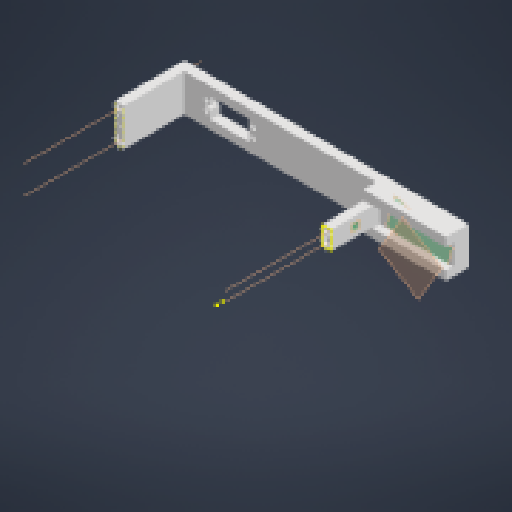
# Autodesk Inventor part: Main Rail
Saved by Autodesk Inventor 2025.2 (Build 292293000, 293)
## iProperties
Created: 2024-11-17
Part Number: Main Rail
Material: Generic
Document SubType Name: Modeling
Designer: JL
Density: 1 g/cm^3
Appearance: Default
Author: JL
Autodesk Inventor part; units mm, degrees
ref_plane "Work Plane1" through (160.0305, 116.6136, -77.6157) normal (0, 0, -1) x (-0.9606716, 0.277687, 0)
ref_plane "Work Plane3" through (116.7456, 115.7996, -51.6157) normal (-1, 0, 0) x (0, 0, 1)
ref_plane "Work Plane2" through (114.2456, 115.7996, -51.6157) normal (-1, 0, 0) x (0, 0, 1)
sketch "Sketch3" plane through (116.7456, 115.7996, -51.6157) normal (-1, 0, 0) x (0, 0, 1)
  circle A0 centre (0, 0) radius 4 construction
  line L0 (-26, 10) -> (0, 10)
  line L1 (0, 10) -> (0, -10)
  line L2 (0, -10) -> (-26, -10)
  line L3 (-26, -10) -> (-26, 10) projected
  point P0 (51.6157, -115.7996)
  constraints: 6 end point, 2 perpendicular, 1 horizontal, 1 midpoint
extrude "Extrusion3" add sketch "Sketch3" along normal blind 10
ref_plane "Work Plane4" through (185.8339, 132.1316, -51.6157) normal (0, 0, 1) x (-0.8564988, 0.516149, 0)
mirror "Mirror1" about plane through (185.8339, 132.1316, -51.6157) normal (0, 0, 1) of "Extrusion3"
sketch "Sketch4" plane through (116.7456, 115.7996, -51.6157) normal (1, 0, 0) x (0, 0, -1)
  circle A0 centre (0, 0) radius 4 projected
  point P0 (-51.6157, -115.7996)
extrude "Extrusion4" cut sketch "Sketch4" against normal up to surface (2.5 mm away)
ref_plane "Work Plane6" through (-26.356, 110.799, -94.8157) normal (0, 0, -1) x (0.8545404, 0.519385, 0)
sketch "Sketch7" plane through (116.7456, 105.7996, -25.6157) normal (0, 0, 1) x (1, 0, 0)
  line L0 (0, 20) -> (0, 0) projected
  line L1 (0, 20) -> (-10, 20) projected
  line L2 (-10, 20) -> (-10, 0) projected
  line L3 (0, 0) -> (-10, 0) projected
  line L4 (0, 10) -> (-10, 10) construction
  line L5 (-5, 10) -> (-5, 0) construction
  point P0 (-116.7456, -105.7996)
  point P1 (-5, 5)
  point P2 (-5, 15)
  constraints: 5 midpoint, 4 end point, 1 symmetric about line
sketch "Sketch11" plane through (-26.356, 110.799, -94.8157) normal (0, 0, -1) x (0.8545404, 0.519385, 0)
  line L0 (4.1262, -15.4557) -> (-6.6251, 2.2333) construction
  line L1 (-6.6251, 2.2333) -> (-41.9176, -19.2173) construction
  line L2 (-41.9176, -19.2173) -> (-31.1663, -36.9063) construction
  line L3 (-31.1663, -36.9063) -> (4.1262, -15.4557) construction
  line L4 (147.168, 71.8939) -> (180.9407, 92.4208) construction
  line L5 (170.553, 109.5116) -> (136.7803, 88.9847) construction
  line L6 (17.8654, -18.8072) -> (-3.2735, 15.9725) construction
  line L7 (-3.2735, 15.9725) -> (-55.6569, -15.8658)
  line L8 (-55.6569, -15.8658) -> (-34.5179, -50.6455) construction
  line L9 (-34.5179, -50.6455) -> (17.8654, -18.8072)
  line L10 (180.9407, 92.4208) -> (198.0315, 102.8085) construction
  line L11 (198.0315, 102.8085) -> (187.4621, 120.1984)
  line L12 (187.6438, 119.8993) -> (170.553, 109.5116) construction
  line L13 (17.8654, -18.8072) -> (203.4072, 93.964)
  line L14 (203.4072, 93.964) -> (198.0315, 102.8085)
  line L15 (187.4621, 120.1984) -> (182.2682, 128.7438)
  line L16 (182.2682, 128.7438) -> (-3.2735, 15.9725)
  circle A0 centre (-27.3984, -22.5044) radius 24.5216 construction
  line L17 (-48.3531, -35.2405) -> (-69.7166, -48.2251) construction
  line L18 (-34.5179, -50.6455) -> (-59.1471, -65.615)
  line L19 (-59.1471, -65.615) -> (-80.2861, -30.8352)
  line L20 (-80.2861, -30.8352) -> (-55.6569, -15.8658)
  line L21 (-42.6046, -19.0497) -> (-6.4575, 2.9203)
  line L22 (-6.4575, 2.9203) -> (4.8131, -15.6233)
  line L23 (4.8131, -15.6233) -> (-31.3339, -37.5933)
  line L24 (-31.3339, -37.5933) -> (-42.6046, -19.0497)
  point P0 (-35.0251, 108.3711)
  dimension "d31" = 10
  dimension "d32" = 20
  dimension "d33" = 25
  dimension "d34" = 0.5
  constraints: 38 end point, 5 perpendicular, 3 collinear, 3 point on line, 1 midpoint, 1 parallel, 9 other
  measures "d31" distance between parallel lines of L3 L9
  measures "d32" distance of L4.end L10.end
  measures "d33" distance of L17.end L17.start
  measures "d34" distance between parallel lines of L1 L21
ref_plane "Work Plane7" through (-30.7879, 116.4111, -84.2157) normal (0, 0, 1) x (0.7646407, 0.6444568, 0)
extrude "Extrusion8" add sketch "Sketch11" against normal up to surface (10.6 mm away)
sketch "Sketch12" plane through (-110.979, 136.1496, -84.2157) normal (0, 0, 1) x (1, 0, 0)
  line L0 (217.7246, -10.35) -> (217.7246, -30.35) projected
  line L1 (307.2462, 0) -> (307.2462, -40.7) projected
  line L2 (0, 0) -> (307.2462, 0) projected
  line L3 (0, -40.7) -> (0, 0) projected
  line L4 (307.2462, -40.7) -> (0, -40.7) projected
  line L5 (217.7246, -10.35) -> (217.7246, 0)
  line L6 (0, 0) -> (307.2462, 0) projected
  line L7 (217.7246, -30.35) -> (217.7246, -40.7)
  point P0 (110.979, -136.1496)
  point P1 (217.7246, 0)
  constraints: 4 end point, 3 point on line, 1 perpendicular
extrude "Extrusion9" add sketch "Sketch12" along normal up to surface (6.6 mm away) contours L5 L2 L1 L4 L7 L0
sketch "Sketch13" plane through (116.7456, 105.7996, -77.6157) normal (0, 0, 1) x (1, 0, 0)
  line L0 (0, 0) -> (-10, 0) projected
  line L1 (-10, 0) -> (-10, -10.35) projected
  line L2 (-10, -10.35) -> (79.5216, -10.35) projected
  line L3 (79.5216, -10.35) -> (79.5216, 30.35) projected
  line L4 (79.5216, 30.35) -> (-10, 30.35) projected
  line L5 (-10, 30.35) -> (-10, 20) projected
  line L6 (0, 20) -> (-10, 20) projected
  line L7 (0, 20) -> (0, 0) projected
  line L8 (0, 20) -> (79.5216, 20)
  line L9 (0, 0) -> (79.5216, 0)
  point P0 (-116.7456, -105.7996)
  constraints: 4 end point, 2 perpendicular, 2 point on line
extrude "Extrusion10" add sketch "Sketch13" along normal blind 7.5 contours L9 L3 L2 L1 L0 | L6 L5 L4 L3 L8
sketch "Sketch14" plane through (-110.979, 136.1496, -84.2157) normal (0, 0, 1) x (1, 0, 0)
  line L0 (0, 0) -> (307.2462, 0) projected
  line L1 (307.2462, -40.7) -> (0, -40.7) projected
  line L2 (0, 0) -> (10, 0)
  line L3 (10, 0) -> (10, -40.7)
  line L4 (10, -40.7) -> (0, -40.7)
  line L5 (0, -40.7) -> (0, 0)
  point P0 (110.979, -136.1496)
  point P1 (10, 0)
  dimension "d41" = 10
  constraints: 8 end point, 2 parallel, 1 horizontal, 1 perpendicular, 1 point on line
  measures "d41" distance between parallel lines of L5 L3
extrude "Extrusion11" add sketch "Sketch14" along normal up to surface (32.6 mm away)
mirror "Mirror2" about plane through (185.8339, 132.1316, -51.6157) normal (0, 0, 1) of "Extrusion11"
sketch "Sketch15" plane through (-110.979, 95.4496, -19.0157) normal (0, 0, 1) x (1, 0, 0)
  line L0 (0, 0) -> (10, 0) construction
  line L1 (5, 0) -> (5, 10) construction
  line L2 (10, 0) -> (10, 40.7) construction
  line L3 (10, 20.35) -> (0, 20.35) construction
  line L4 (0, 40.7) -> (0, 0) construction
  point P0 (110.979, -95.4496)
  point P1 (5, 5)
  point P2 (5, 35.7)
  constraints: 4 end point, 4 midpoint, 1 perpendicular, 1 symmetric about line, 1 vertical
sketch "Sketch17" plane through (116.7456, 105.7996, -25.6157) normal (0, 0, 1) x (1, 0, 0)
  circle A0 centre (-5.0015, 4.9996) radius 2.77 projected
  circle A1 centre (-5.0015, 14.9996) radius 2.77 projected
  point P0 (-116.7456, -105.7996)
ref_plane "Work Plane10" through (108.2326, 107.2877, -33.7157) normal (0, 0, -1) x (0.3976268, 0.9175472, 0)
extrude "Extrusion13" cut sketch "Sketch17" against normal up to surface (8.1 mm away)
sketch "Sketch18" plane through (111.7441, 110.7992, -33.7157) normal (0, 0, 1) x (1, 0, 0)
  circle A0 centre (0, 0) radius 2.77 projected
  circle A1 centre (0, 10) radius 2.77 projected
  point P0 (-111.7441, -110.7992)
  constraints: 2 coincident
hole "Hole2" at (111.7441, 110.7992, -33.7157) at (111.7441, 120.7992, -33.7157) direction (0, 0, -1) diameter 4.3 end through all clearance for "Flat Head Machine Screw" size "M4" standard "Ansi Metric M Profile"
sketch "Sketch19" plane through (-110.979, 95.4496, -19.0157) normal (0, 0, 1) x (1, 0, 0)
  circle A0 centre (4.9984, 35.7) radius 2.77 projected
  circle A1 centre (4.9985, 4.9996) radius 2.77 projected
  point P0 (110.979, -95.4496)
ref_plane "Work Plane11" through (-109.4921, 96.9377, -27.1157) normal (0, 0, -1) x (0.3976268, 0.9175472, 0)
extrude "Extrusion14" cut sketch "Sketch19" against normal up to surface (8.1 mm away)
sketch "Sketch20" plane through (-105.9806, 131.1496, -27.1157) normal (0, 0, 1) x (1, 0, 0)
  circle A0 centre (0, 0) radius 2.77 projected
  circle A1 centre (0, -30.7004) radius 2.77 projected
  circle A2 centre (0, 0) radius 2.77 projected
  point P0 (105.9806, -131.1496)
  constraints: 2 coincident
hole "Hole3" at (-105.9806, 131.1496, -27.1157) at (-105.9805, 100.4492, -27.1157) direction (0, 0, -1) diameter 4.3 end through all clearance for "Flat Head Machine Screw" size "M4" standard "Ansi Metric M Profile"
sketch "Sketch21" plane through (106.7456, 95.4496, -84.2157) normal (0, 0, 1) x (1, 0, 0)
  circle A0 centre (-133.1046, 25.3503) radius 2.77 projected
  circle A1 centre (-133.1016, 15.3494) radius 2.77 projected
  circle A2 centre (-183.4046, 25.3502) radius 2.77 projected
  circle A3 centre (-183.4046, 15.3496) radius 2.77 projected
  point P0 (-106.7456, -95.4496)
ref_plane "Work Plane12" through (-80.4345, 117.0243, -92.3157) normal (0, 0, -1) x (0.6957438, 0.7182901, 0)
extrude "Extrusion15" cut sketch "Sketch21" against normal up to surface (8.1 mm away)
sketch "Sketch22" plane through (-76.659, 120.7998, -92.3157) normal (0, 0, 1) x (1, 0, 0)
  circle A0 centre (0, 0) radius 2.77 projected
  circle A1 centre (0, -10.0006) radius 2.77 projected
  circle A2 centre (50.3, 0.0002) radius 2.77 projected
  circle A3 centre (50.3031, -10.0008) radius 2.77 projected
  point P0 (76.659, -120.7998)
  constraints: 4 coincident
hole "Hole4" at (-76.659, 120.7998, -92.3157) at (-76.659, 110.7992, -92.3157) at (-26.356, 110.799, -92.3157) at (-26.359, 120.8, -92.3157) direction (0, 0, -1) diameter 4.3 end through all clearance for "Flat Head Machine Screw" size "M4" standard "Ansi Metric M Profile"
sketch "Sketch23" plane through (106.7456, 95.4496, -84.2157) normal (0, 0, 1) x (1, 0, 0)
  line L0 (-179.4031, 31.2) -> (-179.4031, 9.5) construction
  line L1 (-179.4031, 22.35) -> (-184.1531, 22.35)
  line L2 (-184.1531, 22.35) -> (-184.1531, 18.35)
  line L3 (-184.1531, 18.35) -> (-179.4031, 18.35)
  line L4 (-179.4031, 18.35) -> (-179.4031, 22.35)
  point P0 (-106.7456, -95.4496)
  point P1 (-179.4031, 20.35)
  dimension "d73" = 4.75
  dimension "d74" = 4
  constraints: 8 end point, 2 midpoint, 2 parallel, 1 horizontal, 1 perpendicular, 1 point on line
  measures "d73" distance of L3.end L2.end
  measures "d74" distance of L2.end L1.end
extrude "Extrusion16" cut sketch "Sketch23" against normal through all
thicken "Thicken1" operation cut thickness 1 both sides no extend neighbours no toward (0, 1, 0) faces at (169.76, 125.7996, -72.6157) (169.76, 119.133, -77.6157) (169.76, 105.7996, -75.1157)
body "Solid1"
